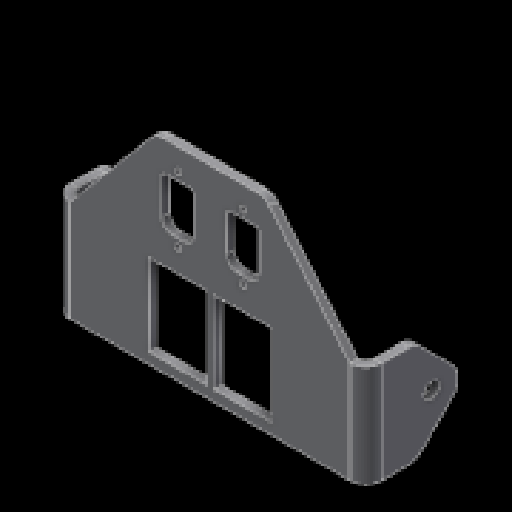
# Autodesk Inventor part: PowerHubEndPanel
Saved by Autodesk Inventor 2025.2 (Build 292293000, 293)
## iProperties
Created: 2026-06-06
Part Number: PowerHubEndPanel
Material: Generic
Document SubType Name: Sheet Metal
Designer: valer
Density: 1 g/cm^3
Appearance: Default
Sheet Metal Rule: Default
Author: valer
Autodesk Inventor part; units mm, degrees
ref_plane "YZ Plane" through (0, 0, 0) normal (1, 0, 0) x (0, 1, 0)
ref_plane "XZ Plane" through (0, 0, 0) normal (0, 1, 0) x (-1, 0, 0)
ref_plane "XY Plane" through (0, 0, 0) normal (0, 0, 1) x (1, 0, 0)
sketch "Base" plane through (0, 0, 0) normal (0, 0, 1) x (1, 0, 0)
  line L0 (-44.957, 34.75) -> (-28.957, 34.75) construction
  line L1 (-28.957, 34.75) -> (-28.957, 0.75) construction
  line L2 (-28.957, 0.75) -> (-44.957, 0.75) construction
  line L3 (-44.957, 0.75) -> (-44.957, 34.75) construction
  line L4 (-49.276, -3.25) -> (-24.638, -3.25) construction
  line L5 (-24.638, -3.25) -> (-24.638, -34.75) construction
  line L6 (-24.638, -34.75) -> (-49.276, -34.75) construction
  line L7 (-49.276, -34.75) -> (-49.276, -3.25) construction
  line L8 (-36.957, 0.75) -> (-36.957, -3.25) construction
  line L9 (-20.319, 0.75) -> (-20.319, 34.75) construction
  line L10 (-20.319, 34.75) -> (-4.319, 34.75) construction
  line L11 (-4.319, 34.75) -> (-4.319, 0.75) construction
  line L12 (-4.319, 0.75) -> (-20.319, 0.75) construction
  line L13 (-24.638, -3.25) -> (0, -3.25) construction
  line L14 (-24.638, -34.75) -> (-24.638, -3.25) construction
  line L15 (0, -3.25) -> (0, -34.75) construction
  line L16 (0, -34.75) -> (-24.638, -34.75) construction
  line L17 (4.319, 0.75) -> (4.319, 34.75) construction
  line L18 (4.319, 34.75) -> (20.319, 34.75) construction
  line L19 (20.319, 34.75) -> (20.319, 0.75) construction
  line L20 (20.319, 0.75) -> (4.319, 0.75) construction
  line L21 (0, -3.25) -> (24.638, -3.25) construction
  line L22 (0, -34.75) -> (0, -3.25) construction
  line L23 (24.638, -3.25) -> (24.638, -34.75) construction
  line L24 (24.638, -34.75) -> (0, -34.75) construction
  line L25 (28.957, 0.75) -> (28.957, 34.75) construction
  line L26 (28.957, 34.75) -> (44.957, 34.75) construction
  line L27 (44.957, 34.75) -> (44.957, 0.75) construction
  line L28 (44.957, 0.75) -> (28.957, 0.75) construction
  line L29 (24.638, -3.25) -> (49.276, -3.25) construction
  line L30 (24.638, -34.75) -> (24.638, -3.25) construction
  line L31 (49.276, -3.25) -> (49.276, -34.75) construction
  line L32 (49.276, -34.75) -> (24.638, -34.75) construction
  line L33 (-53.276, 38.75) -> (53.276, 38.75)
  line L34 (53.276, 38.75) -> (53.276, -38.75)
  line L35 (53.276, -38.75) -> (-53.276, -38.75)
  line L36 (-53.276, -38.75) -> (-53.276, 38.75)
  line L37 (0, -54.25) -> (0, 54.25)
  line L38 (-53.276, 38.75) -> (53.276, -38.75) construction
  point P0 (-12.319, 0.75)
  point P1 (-12.319, -3.25)
  point P2 (12.319, 0.75)
  point P3 (12.319, -3.25)
  point P4 (36.957, 0.75)
  point P5 (36.957, -3.25)
  point P6 (0, 0)
  point P7 (0, 0)
  dimension "d103" = 16
  dimension "d104" = 34
  dimension "d105" = 24.638
  dimension "d106" = 31.5
  dimension "d107" = 4
  dimension "d110" = 24.638
  dimension "d125" = 4
  dimension "d126" = 4
  dimension "d131" = 4
  dimension "d132" = 4
  measures "d103" distance of L0.start L0.end
  measures "d104" distance of L0.end L1.end
  measures "d105" distance of L5.end L6.end
  measures "d106" distance of L4.end L5.end
  measures "d107" distance between parallel lines of L4 L2
  measures "d110" distance of L2.end L9.start
  measures "d125" distance between parallel lines of L36 L7
  measures "d126" distance between parallel lines of L34 L31
  measures "d131" distance between parallel lines of L33 L26
  measures "d132" distance between parallel lines of L35 L32
extrude "Plate1" add sketch "Base" along normal blind 3.048
sketch "Instruments" plane through (0, 0, 0) normal (0, 0, -1) x (-1, 0, 0)
  circle A0 centre (-37.174, 14.35) radius 2.5 construction
  circle A1 centre (-37.174, 21.35) radius 2.5 construction
  arc A2 (-43.074, 12.4) -> (-39.274, 8.6) centre (-39.274, 12.4) ccw construction
  line L0 (-39.274, 8.6) -> (-35.074, 8.6) construction
  arc A3 (-35.074, 8.6) -> (-31.274, 12.4) centre (-35.074, 12.4) ccw construction
  line L1 (-31.274, 12.4) -> (-31.274, 26.1) construction
  arc A4 (-31.274, 26.1) -> (-32.274, 27.1) centre (-32.274, 26.1) ccw construction
  line L2 (-32.274, 27.1) -> (-42.074, 27.1) construction
  arc A5 (-42.074, 27.1) -> (-43.074, 26.1) centre (-42.074, 26.1) ccw construction
  line L3 (-43.074, 26.1) -> (-43.074, 12.4) construction
  circle A6 centre (-12.474, 14.35) radius 2.5 construction
  circle A7 centre (-12.474, 21.35) radius 2.5 construction
  arc A8 (-18.374, 12.4) -> (-14.574, 8.6) centre (-14.574, 12.4) ccw construction
  line L4 (-14.574, 8.6) -> (-10.374, 8.6) construction
  arc A9 (-10.374, 8.6) -> (-6.574, 12.4) centre (-10.374, 12.4) ccw construction
  line L5 (-6.574, 12.4) -> (-6.574, 26.1) construction
  arc A10 (-6.574, 26.1) -> (-7.574, 27.1) centre (-7.574, 26.1) ccw construction
  line L6 (-7.574, 27.1) -> (-17.374, 27.1) construction
  arc A11 (-17.374, 27.1) -> (-18.374, 26.1) centre (-17.374, 26.1) ccw construction
  line L7 (-18.374, 26.1) -> (-18.374, 12.4) construction
  circle A12 centre (12.226, 14.35) radius 2.5 construction
  circle A13 centre (12.226, 21.35) radius 2.5 construction
  arc A14 (6.326, 12.4) -> (10.126, 8.6) centre (10.126, 12.4) ccw construction
  line L8 (10.126, 8.6) -> (14.326, 8.6) construction
  arc A15 (14.326, 8.6) -> (18.126, 12.4) centre (14.326, 12.4) ccw construction
  line L9 (18.126, 12.4) -> (18.126, 26.1) construction
  arc A16 (18.126, 26.1) -> (17.126, 27.1) centre (17.126, 26.1) ccw construction
  line L10 (17.126, 27.1) -> (7.326, 27.1) construction
  arc A17 (7.326, 27.1) -> (6.326, 26.1) centre (7.326, 26.1) ccw construction
  line L11 (6.326, 26.1) -> (6.326, 12.4) construction
  circle A18 centre (36.926, 14.35) radius 2.5 construction
  circle A19 centre (36.926, 21.35) radius 2.5 construction
  arc A20 (31.026, 12.4) -> (34.826, 8.6) centre (34.826, 12.4) ccw construction
  line L12 (34.826, 8.6) -> (39.026, 8.6) construction
  arc A21 (39.026, 8.6) -> (42.826, 12.4) centre (39.026, 12.4) ccw construction
  line L13 (42.826, 12.4) -> (42.826, 26.1) construction
  arc A22 (42.826, 26.1) -> (41.826, 27.1) centre (41.826, 26.1) ccw construction
  line L14 (41.826, 27.1) -> (32.026, 27.1) construction
  arc A23 (32.026, 27.1) -> (31.026, 26.1) centre (32.026, 26.1) ccw construction
  line L15 (31.026, 26.1) -> (31.026, 12.4) construction
  line L16 (-43.8196, -7.45) -> (-30.5284, -7.45) construction
  line L17 (-30.5284, -7.45) -> (-30.5284, -30.45) construction
  line L18 (-30.5284, -30.45) -> (-43.8196, -30.45) construction
  line L19 (-43.8196, -30.45) -> (-43.8196, -7.45) construction
  line L20 (-26.379, -3.6) -> (-47.969, -3.6) construction
  line L21 (-47.969, -3.6) -> (-47.969, -34.3) construction
  line L22 (-47.969, -34.3) -> (-26.379, -34.3) construction
  line L23 (-26.379, -34.3) -> (-26.379, -3.6) construction
  line L24 (-19.1196, -7.45) -> (-5.8284, -7.45) construction
  line L25 (-5.8284, -7.45) -> (-5.8284, -30.45) construction
  line L26 (-5.8284, -30.45) -> (-19.1196, -30.45) construction
  line L27 (-19.1196, -30.45) -> (-19.1196, -7.45) construction
  line L28 (-1.679, -3.6) -> (-23.269, -3.6) construction
  line L29 (-23.269, -3.6) -> (-23.269, -34.3) construction
  line L30 (-23.269, -34.3) -> (-1.679, -34.3) construction
  line L31 (-1.679, -34.3) -> (-1.679, -3.6) construction
  line L32 (5.5804, -7.45) -> (18.8716, -7.45) construction
  line L33 (18.8716, -7.45) -> (18.8716, -30.45) construction
  line L34 (18.8716, -30.45) -> (5.5804, -30.45) construction
  line L35 (5.5804, -30.45) -> (5.5804, -7.45) construction
  line L36 (23.021, -3.6) -> (1.431, -3.6) construction
  line L37 (1.431, -3.6) -> (1.431, -34.3) construction
  line L38 (1.431, -34.3) -> (23.021, -34.3) construction
  line L39 (23.021, -34.3) -> (23.021, -3.6) construction
  line L40 (30.2804, -7.45) -> (43.5716, -7.45) construction
  line L41 (43.5716, -7.45) -> (43.5716, -30.45) construction
  line L42 (43.5716, -30.45) -> (30.2804, -30.45) construction
  line L43 (30.2804, -30.45) -> (30.2804, -7.45) construction
  line L44 (47.721, -3.6) -> (26.131, -3.6) construction
  line L45 (26.131, -3.6) -> (26.131, -34.3) construction
  line L46 (26.131, -34.3) -> (47.721, -34.3) construction
  line L47 (47.721, -34.3) -> (47.721, -3.6) construction
  line L48 (-42.074, 27.35) -> (-32.274, 27.35)
  arc A24 (-31.024, 26.1) -> (-32.274, 27.35) centre (-32.274, 26.1) ccw
  line L49 (-31.024, 26.1) -> (-31.024, 12.4)
  arc A25 (-35.074, 8.35) -> (-31.024, 12.4) centre (-35.074, 12.4) ccw
  line L50 (-35.074, 8.35) -> (-39.274, 8.35)
  arc A26 (-43.324, 12.4) -> (-39.274, 8.35) centre (-39.274, 12.4) ccw
  line L51 (-43.324, 12.4) -> (-43.324, 26.1)
  arc A27 (-42.074, 27.35) -> (-43.324, 26.1) centre (-42.074, 26.1) ccw
  line L52 (-17.374, 27.35) -> (-7.574, 27.35)
  arc A28 (-6.324, 26.1) -> (-7.574, 27.35) centre (-7.574, 26.1) ccw
  line L53 (-6.324, 26.1) -> (-6.324, 12.4)
  arc A29 (-10.374, 8.35) -> (-6.324, 12.4) centre (-10.374, 12.4) ccw
  line L54 (-10.374, 8.35) -> (-14.574, 8.35)
  arc A30 (-18.624, 12.4) -> (-14.574, 8.35) centre (-14.574, 12.4) ccw
  line L55 (-18.624, 12.4) -> (-18.624, 26.1)
  arc A31 (-17.374, 27.35) -> (-18.624, 26.1) centre (-17.374, 26.1) ccw
  line L56 (7.326, 27.35) -> (17.126, 27.35)
  arc A32 (18.376, 26.1) -> (17.126, 27.35) centre (17.126, 26.1) ccw
  line L57 (18.376, 26.1) -> (18.376, 12.4)
  arc A33 (14.326, 8.35) -> (18.376, 12.4) centre (14.326, 12.4) ccw
  line L58 (14.326, 8.35) -> (10.126, 8.35)
  arc A34 (6.076, 12.4) -> (10.126, 8.35) centre (10.126, 12.4) ccw
  line L59 (6.076, 12.4) -> (6.076, 26.1)
  arc A35 (7.326, 27.35) -> (6.076, 26.1) centre (7.326, 26.1) ccw
  line L60 (32.026, 27.35) -> (41.826, 27.35)
  arc A36 (43.076, 26.1) -> (41.826, 27.35) centre (41.826, 26.1) ccw
  line L61 (43.076, 26.1) -> (43.076, 12.4)
  arc A37 (39.026, 8.35) -> (43.076, 12.4) centre (39.026, 12.4) ccw
  line L62 (39.026, 8.35) -> (34.826, 8.35)
  arc A38 (30.776, 12.4) -> (34.826, 8.35) centre (34.826, 12.4) ccw
  line L63 (30.776, 12.4) -> (30.776, 26.1)
  arc A39 (32.026, 27.35) -> (30.776, 26.1) centre (32.026, 26.1) ccw
  line L64 (47.971, -3.35) -> (25.881, -3.35)
  line L65 (25.881, -3.35) -> (25.881, -34.55)
  line L66 (25.881, -34.55) -> (47.971, -34.55)
  line L67 (47.971, -34.55) -> (47.971, -3.35)
  line L68 (1.181, -3.35) -> (23.271, -3.35)
  line L69 (23.271, -3.35) -> (23.271, -34.55)
  line L70 (23.271, -34.55) -> (1.181, -34.55)
  line L71 (1.181, -34.55) -> (1.181, -3.35)
  line L72 (-23.519, -3.35) -> (-1.429, -3.35)
  line L73 (-1.429, -3.35) -> (-1.429, -34.55)
  line L74 (-1.429, -34.55) -> (-23.519, -34.55)
  line L75 (-23.519, -34.55) -> (-23.519, -3.35)
  line L76 (-48.219, -3.35) -> (-26.129, -3.35)
  line L77 (-26.129, -3.35) -> (-26.129, -34.55)
  line L78 (-26.129, -34.55) -> (-48.219, -34.55)
  line L79 (-48.219, -34.55) -> (-48.219, -3.35)
  circle A40 centre (36.926, 30.35) radius 1.55 construction
  circle A41 centre (36.926, 5.35) radius 1.55 construction
  circle A42 centre (12.226, 5.35) radius 1.55 construction
  circle A43 centre (12.226, 30.35) radius 1.55 construction
  circle A44 centre (-12.474, 30.35) radius 1.55 construction
  circle A45 centre (-12.474, 5.35) radius 1.55 construction
  circle A46 centre (-37.174, 30.35) radius 1.55 construction
  circle A47 centre (-37.174, 5.35) radius 1.55 construction
  circle A48 centre (-37.174, 30.35) radius 1.25
  circle A49 centre (-12.474, 30.35) radius 1.25
  circle A50 centre (12.226, 30.35) radius 1.25
  circle A51 centre (36.926, 30.35) radius 1.25
  circle A52 centre (-37.174, 5.35) radius 1.25
  circle A53 centre (-12.474, 5.35) radius 1.25
  circle A54 centre (12.226, 5.35) radius 1.25
  circle A55 centre (36.926, 5.35) radius 1.25
  point P0 (0, 0)
  dimension "d134" = 0.25
  dimension "d135" = 0.25
  dimension "d136" = 0.25
  dimension "d137" = 0.25
  dimension "d138" = 0.25
  dimension "d139" = 0.25
  dimension "d140" = 0.25
  dimension "d141" = 0.25
  dimension "d144" = 2.5
  constraints: 64 end point, 32 point on circle, 24 centre point, 8 coincident, 7 equal radius, 40 other
  measures "d134" distance between parallel lines of L2 L48
  measures "d135" distance between parallel lines of L6 L52
  measures "d136" distance between parallel lines of L10 L56
  measures "d137" distance between parallel lines of L14 L60
  measures "d138" distance between parallel lines of L47 L67
  measures "d139" distance between parallel lines of L36 L68
  measures "d140" distance between parallel lines of L28 L72
  measures "d141" distance between parallel lines of L20 L76
  measures "d144" diameter of A48
extrude "InstrumentsFeature" cut sketch "Instruments" against normal blind 3.048 contours L52 A28 L53 A29 L54 A30 L55 A31 | L56 A32 L57 A33 L58 A34 L59 A35 | L68 L69 L70 L71 | L72 L73 L74 L75 | A49 | A50 | A53 | A54
sketch "Taper" plane through (0, 0, 3.048) normal (0, 0, 1) x (1, 0, 0)
  circle A0 centre (12.474, 30.35) radius 1.25 projected
  line L0 (1.429, -34.55) -> (1.429, -3.35) projected
  line L1 (1.429, -3.35) -> (23.519, -3.35) projected
  line L2 (23.519, -3.35) -> (23.519, -34.55) projected
  line L3 (23.519, -34.55) -> (1.429, -34.55) projected
  arc A1 (-18.376, 12.4) -> (-14.326, 8.35) centre (-14.326, 12.4) ccw projected
  line L4 (-18.376, 12.4) -> (-18.376, 26.1) projected
  arc A2 (-17.126, 27.35) -> (-18.376, 26.1) centre (-17.126, 26.1) ccw projected
  line L5 (-17.126, 27.35) -> (-7.326, 27.35) projected
  arc A3 (-6.076, 26.1) -> (-7.326, 27.35) centre (-7.326, 26.1) ccw projected
  line L6 (-6.076, 26.1) -> (-6.076, 12.4) projected
  arc A4 (-10.126, 8.35) -> (-6.076, 12.4) centre (-10.126, 12.4) ccw projected
  line L7 (-10.126, 8.35) -> (-14.326, 8.35) projected
  circle A5 centre (-12.226, 30.35) radius 1.25 projected
  circle A6 centre (12.474, 5.35) radius 1.25 projected
  line L8 (-23.271, -34.55) -> (-23.271, -3.35) projected
  line L9 (-23.271, -3.35) -> (-1.181, -3.35) projected
  line L10 (-1.181, -3.35) -> (-1.181, -34.55) projected
  line L11 (-1.181, -34.55) -> (-23.271, -34.55) projected
  arc A7 (6.324, 12.4) -> (10.374, 8.35) centre (10.374, 12.4) ccw projected
  line L12 (6.324, 12.4) -> (6.324, 26.1) projected
  arc A8 (7.574, 27.35) -> (6.324, 26.1) centre (7.574, 26.1) ccw projected
  line L13 (7.574, 27.35) -> (17.374, 27.35) projected
  arc A9 (18.624, 26.1) -> (17.374, 27.35) centre (17.374, 26.1) ccw projected
  line L14 (18.624, 26.1) -> (18.624, 12.4) projected
  arc A10 (14.574, 8.35) -> (18.624, 12.4) centre (14.574, 12.4) ccw projected
  line L15 (14.574, 8.35) -> (10.374, 8.35) projected
  circle A11 centre (-12.226, 5.35) radius 1.25 projected
  line L16 (-53.276, -38.75) -> (-53.276, 38.75) projected
  line L17 (53.276, -38.75) -> (-53.276, -38.75) projected
  line L18 (53.276, 38.75) -> (53.276, -38.75) projected
  line L19 (-53.276, 38.75) -> (53.276, 38.75) projected
  line L20 (0, -54.25) -> (0, 54.25) construction
  line L21 (-53.276, -38.75) -> (53.276, -38.75) projected
  line L22 (-53.276, -38.75) -> (-53.276, 0)
  line L23 (-53.276, 0) -> (-26.143, 38.75)
  line L24 (53.276, 38.75) -> (-53.276, 38.75) projected
  line L25 (-74.5864, 0) -> (74.5864, 0) construction
  line L26 (53.276, -38.75) -> (53.276, 0)
  line L27 (53.276, 0) -> (26.143, 38.75)
  point P0 (0, 0)
  dimension "d159" = 55
  constraints: 8 end point, 2 point on line, 2 symmetric about line, 1 midpoint
  measures "d159" angle of L25 L23
extrude "TaperFeature" cut sketch "Taper" against normal blind 3.048 contours L16 L19 L23 | L27 L19 L18
sketch "Sketch10" plane through (-56.324, 0, -3.048) normal (-1, 0, 0) x (0, -1, 0)
  line L0 (38.75, 0) -> (0, 0)
  line L1 (0, 0) -> (0, -28.904)
  line L2 (0, -28.904) -> (38.75, -28.904)
  line L3 (38.75, -28.904) -> (38.75, 0)
  constraints: 6 end point, 1 horizontal, 1 perpendicular, 1 vertical
edge flange "MountFeature" height 35 angle 90 thickness 3.048 bend radius 3.048 thickness toward (-1, 0, 0) relief straight relief width 3.048 relief depth 1.524 corner gap 3.048 corner form 0 edges at (-53.276, -19.375, 0) (53.276, -19.375, 0) wall of the first edge with corners at (-56.324, -38.75, -3.048) (-56.324, 0, -3.048) (-56.324, 0, -31.952) (-56.324, -38.75, -31.952)
bend "Bend1"
corner "Corner1"
chamfer "MountChamfersFeature" distance 16 angle 45 4 edges at (57.848, -38.75, -31.952) (-57.848, -38.75, -31.952) (57.848, 0, -31.952) (-57.848, 0, -31.952)
fillet "MountFilletsFeature" radius 6 8 edges at (57.848, -38.75, -15.952) (57.848, -22.75, -31.952) (-57.848, -38.75, -15.952) (-57.848, -22.75, -31.952) (57.848, -16, -31.952) (57.848, 0, -15.952) (-57.848, -16, -31.952) (-57.848, 0, -15.952)
sketch "Sketch12" plane through (-59.372, -38.75, -3.048) normal (-1, 0, 0) x (0, 0, 1)
  circle A0 centre (-18.904, -19.9878) radius 3 projected
  line L0 (-18.904, -19.9878) -> (-18.904, 32.75)
  line L1 (-27.1466, 24.5074) -> (-14.6614, 36.9926) projected
  circle A1 centre (-18.904, 20.2647) radius 3
  line L2 (-28.904, 18.4853) -> (-28.904, 20.2647) projected
  line L3 (-18.904, 20.2647) -> (-28.904, 20.2647)
  point P0 (3.048, 38.75)
  constraints: 4 end point, 2 point on line, 1 centre point, 1 equal radius, 1 perpendicular, 1 vertical
extrude "Cut3" cut sketch "Sketch12" against normal through all contours A1 L3 L0 | L0 A1 | L3 A1 L0
fillet "Fillet3" radius 6 2 edges at (-26.143, 38.75, 1.524) (26.143, 38.75, 1.524)
body "Solid3"
